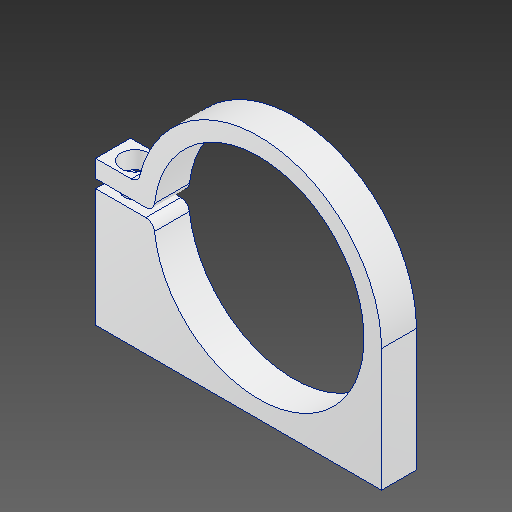
# Autodesk Inventor part: MotorCircularClamp
Saved by Autodesk Inventor 2021 (Build 250183000, 183)
## iProperties
Created: 2021-03-10
Part Number: MotorCircularClamp
Material: Aluminum 6061
Document SubType Name: Modeling
Designer: M3rob
Density: 2.7 g/cm^3
Appearance: Aluminum - Flat
Mass: 98.181 g
Surface Area: 163.009 cm^2
Volume: 36.3633 cm^3
Author: M3rob
Autodesk Inventor part; units mm, degrees
ref_plane "YZ Plane" through (0, 0, 0) normal (1, 0, 0) x (0, 1, 0)
ref_plane "XZ Plane" through (0, 0, 0) normal (0, 1, 0) x (-1, 0, 0)
ref_plane "XY Plane" through (0, 0, 0) normal (0, 0, 1) x (1, 0, 0)
sketch "Sketch1" plane through (0, 0, 0) normal (0, 0, 1) x (1, 0, 0)
  arc A0 (-37.9732, -4.3973) -> (-37.9732, 4.3973) centre (0, 0) ccw
  arc A1 (44.577, 0) -> (-43.3532, 10.3736) centre (0, 0) ccw
  line L0 (-46.441, 7.9375) -> (-46.695, 7.9375)
  line L1 (-59.395, 7.9375) -> (-59.395, 1.5875)
  line L2 (-59.395, 1.5875) -> (-41.1272, 1.5875)
  line L3 (0, 38.227) -> (0, 44.577) construction
  line L4 (-61.9125, 7.9375) -> (-61.9125, 1.5875) construction
  line L5 (-59.395, -1.5875) -> (-59.395, -44.577)
  line L6 (-59.395, -44.577) -> (44.577, -44.577)
  line L7 (44.577, -44.577) -> (44.577, 0)
  line L8 (-59.395, -1.5875) -> (-41.1272, -1.5875)
  arc A2 (-38.194, 1.5875) -> (-38.194, -1.5875) centre (0, 0) ccw construction
  line L9 (-56.22, 7.9375) -> (-56.22, -1.5875) construction
  line L10 (-46.695, 7.9375) -> (-46.695, -1.5875) construction
  line L11 (-51.4575, 7.9375) -> (-51.4575, 1.5875) construction
  line L12 (-51.4575, 1.5875) -> (-51.4575, -1.5875) construction
  line L13 (-51.4575, 7.9375) -> (-56.22, 7.9375)
  line L14 (-56.22, 7.9375) -> (-59.395, 7.9375)
  line L15 (-46.695, 7.9375) -> (-51.4575, 7.9375)
  line L16 (0, -38.227) -> (0, -44.577) construction
  arc A3 (-37.9732, -4.3973) -> (-41.1272, -1.5875) centre (-41.1272, -4.7625) ccw
  arc A4 (-41.1272, 1.5875) -> (-37.9732, 4.3973) centre (-41.1272, 4.7625) ccw
  arc A5 (-46.441, 7.9375) -> (-43.3532, 10.3736) centre (-46.441, 11.1125) ccw
  point P0 (-43.8646, 7.9375)
  point P1 (-51.4575, 0)
  dimension "d0" = 76.454
  dimension "d1" = 6.35
  dimension "d2" = 9.525
  dimension "d3" = 3.175
  dimension "d4" = 3.175
  dimension "d5" = 6.35
  dimension "d7" = 3.175
  dimension "d8" = 3.175
  dimension "d38" = 0.254
  constraints: 34 end point, 19 point on circle, 13 point on line, 12 perpendicular, 7 tangent, 6 centre point, 5 horizontal, 2 equal length, 2 horizontal alignment, 2 vertical, 1 coincident, 1 concentric, 1 equal radius, 1 midpoint, 1 vertical alignment, 1 other
  measures "d0" diameter of A0
  measures "d1" radial gap between concentric circles of A1 A0
  measures "d2" distance between parallel lines of L9 L10
  measures "d3" distance between parallel lines of L1 L9
  measures "d4" distance between parallel lines of L8 L2
  measures "d5" distance from line of L2 point (-43.865, 7.937)
  measures "d7" radius of A5
  measures "d8" radius of A3
  measures "d38" distance of L0.start L0.end
extrude "Extrusion1" add sketch "Sketch1" along normal mid plane 12.7
sketch "Sketch2" plane through (-59.395, 7.9375, 6.35) normal (0, 1, 0) x (1, 0, 0)
  point P0 (59.395, 6.35)
  point P1 (7.9375, 6.35)
  point P2 (7.9375, 6.35)
  point P3 (7.9375, 6.35)
hole "Hole1" at (-51.4575, 7.9375, 0) direction (0, -1, 0) diameter 10.0838 depth 6.35 clearance for "Flat Head Machine Screw (82)" size "3/8" standard "Ansi Unified Screw Threads"
sketch "Sketch3" plane through (-59.395, -1.5875, 6.35) normal (0, 1, 0) x (1, 0, 0)
  arc A0 (12.954, 6.8555) -> (12.954, 5.8445) centre (7.9375, 6.35) ccw projected
  point P0 (59.395, 6.35)
hole "Hole2" at (-51.4575, -1.5875, 0) direction (0, -1, 0) diameter 7.7978 depth 27.0002 tip angle 118 thread size "3/8-16 UNC" class "2B" standard "ANSI Unified Screw Threads"
sketch "Sketch4" plane through (-59.395, -44.577, 6.35) normal (0, -1, 0) x (1, 0, 0)
  line L0 (103.972, -12.7) -> (103.972, 0) construction
  line L1 (21.4217, -12.7) -> (21.4217, 0) construction
  line L2 (21.4217, -6.35) -> (15.0717, -6.35) construction
  line L3 (103.972, -6.35) -> (97.622, -6.35) construction
  dimension "d29" = 6.35
  dimension "d30" = 6.35
  constraints: 4 end point, 2 coincident, 2 horizontal, 2 midpoint
  measures "d29" distance of L2.start L2.end
  measures "d30" distance of L3.start L3.end
hole "Hole3" at (-44.3232, -44.577, 0) at (38.227, -44.577, 0) direction (0, 1, 0) diameter 7.7978 depth 27.0002 tip angle 118 thread size "3/8-16 UNC" class "2B" standard "ANSI Unified Screw Threads"
body "Solid1"
